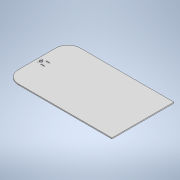
# Autodesk Inventor part: щиток
Saved by Autodesk Inventor 2021.1 (Build 251245010, 245A)
## iProperties
Created: 2023-04-14
Part Number: щиток
Material: Типовые
Document SubType Name: Modeling
Designer: User
Density: 1 g/cm^3
Appearance: По умолчанию
Author: User
Autodesk Inventor part; units mm, degrees
ref_plane "YZ Plane" through (0, 0, 0) normal (1, 0, 0) x (0, 1, 0)
ref_plane "XZ Plane" through (0, 0, 0) normal (0, 1, 0) x (-1, 0, 0)
ref_plane "XY Plane" through (0, 0, 0) normal (0, 0, 1) x (1, 0, 0)
sketch "Эскиз1" plane through (0, 0, 0) normal (0, 1, 0) x (-1, 0, 0)
  ellipse E0 centre (0, 0) end of major axis (0, -190) minor radius 325
  line L0 (0, 190) -> (-325, 190)
  line L1 (-325, 190) -> (-325, -190)
  line L2 (-325, -190) -> (0, -190)
  line L3 (0, -190) -> (0, 190)
  line L4 (0, 190) -> (325, 190)
  line L5 (325, 190) -> (325, -190)
  line L6 (325, -190) -> (0, -190)
  line L7 (0, -190) -> (0, 190)
  point P0 (0, -190)
  dimension "d0" = 325
  dimension "d1" = 190
  constraints: 16 end point, 4 horizontal, 4 parallel, 2 perpendicular, 2 vertical, 1 coincident, 1 vertical alignment, 2 other
extrude "Выдавливание1" add sketch "Эскиз1" along normal blind 6
fillet "Сопряжение1" radius 75 2 edges at (-325, 3, -190) (-325, 3, 190)
sketch "Эскиз2" plane through (0, 0, 0) normal (0, -1, 0) x (1, 0, 0)
  line L0 (-325, 0) -> (325, 0) construction
  line L1 (325, 190) -> (325, -190) projected
  line L2 (-325, 25) -> (-295, 14.0809)
  line L3 (-295, 14.0809) -> (97.2224, 27.7776)
  line L4 (97.2224, 27.7776) -> (125, 0)
  line L5 (-325, -115) -> (-325, 115) projected
  line L6 (-325, -25) -> (-295, -14.0809)
  line L7 (-295, -14.0809) -> (97.2224, -27.7776)
  line L8 (97.2224, -27.7776) -> (125, 0)
  line L9 (-325, 115) -> (-325, -115)
  line L10 (-260, 60) -> (-190, 60)
  line L11 (-190, 60) -> (-190, 130)
  line L12 (-190, 130) -> (-260, 130)
  line L13 (-260, 130) -> (-260, 60)
  line L14 (-190, 60) -> (-175.5025, 95)
  line L15 (-175.5025, 95) -> (-190, 130)
  line L16 (-218.335, 0) -> (-218.335, 60) construction
  line L17 (-250, 190) -> (325, 190) projected
  line L18 (-250, 190) -> (325, 190) projected
  line L19 (-250, 190) -> (-331.0569, 190) construction
  line L20 (-218.335, 130) -> (-218.335, 190) construction
  arc A0 (-250, 190) -> (-325, 115) centre (-250, 115) ccw projected
  line L21 (-175.5025, 51.7755) -> (-260, 130) construction
  line L22 (-260, 60) -> (-175.5025, 138.2245) construction
  circle A1 centre (-222.1933, 95) radius 14.4069 construction
  line L23 (-187.9955, 133) -> (-263, 133)
  line L24 (-263, 133) -> (-263, 57)
  line L25 (-263, 57) -> (-187.9955, 57)
  line L26 (-187.9955, 133) -> (-172.2553, 95)
  line L27 (-172.2553, 95) -> (-187.9955, 57)
  line L28 (-260, 95) -> (-253, 95)
  circle A2 centre (-253, 95) radius 5
  circle A3 centre (-253, 96.8516) radius 0.6666
  circle A4 centre (-253, 93.1484) radius 0.6666
  dimension "d5" = 45
  dimension "d8" = 133
  dimension "d9" = 25
  dimension "d10" = 70
  dimension "d11" = 30
  dimension "d12" = 135
  dimension "d13" = 70
  dimension "d15" = 60
  dimension "d16" = 3
  dimension "d17" = 3
  dimension "d20" = 7
  dimension "d21" = 10
  dimension "d27" = 200
  constraints: 50 end point, 9 point on line, 6 symmetric about line, 4 centre point, 4 equal length, 3 horizontal, 3 midpoint, 3 parallel, 3 perpendicular, 2 collinear, 1 coincident, 4 other
  measures "d5" angle of L4 L0
  measures "d8" angle of L4 L3
  measures "d9" distance from line of L2.start L0
  measures "d10" angle of L5 L2
  measures "d11" distance from line of L5 L2.end
  measures "d12" angle of L15 L14
  measures "d13" distance of L11.end L12.end
  measures "d15" distance from line of A0.centre L11
  measures "d16" distance between parallel lines of L26 L15
  measures "d17" distance between parallel lines of L23 L12
  measures "d20" distance from line of L13 L28.end
  measures "d21" diameter of A2
  measures "d27" distance from line of L1 L4.end
extrude "Выдавливание2" cut sketch "Эскиз2" against normal blind 0.5
sketch "Эскиз3" plane through (0, 0, 0) normal (0, -1, 0) x (1, 0, 0)
  line L0 (-295, -14.0809) -> (-325, -25) projected
  circle A0 centre (-300.125, 0) radius 8.5
  line L1 (97.2224, -27.7776) -> (-295, -14.0809) projected
  line L2 (-295, -14.0809) -> (-300.125, 0) construction
  circle A1 centre (-305.205, -14.48) radius 1.6
  line L3 (-325, -25) -> (-325, 25) projected
  line L4 (-325, 0) -> (327.0887, 0) construction
  line L5 (-308.505, -17.78) -> (-264.055, -17.78)
  line L6 (-264.055, -17.78) -> (-264.055, 17.78)
  line L7 (-264.055, 17.78) -> (-308.505, 17.78)
  line L8 (-308.505, 17.78) -> (-308.505, -17.78)
  line L9 (-264.055, -17.78) -> (-280.3762, 0) construction
  line L10 (-264.055, 17.78) -> (-280.3762, 0) construction
  line L11 (-264.055, 17.78) -> (-285.037, 17.78)
  line L12 (-285.037, 17.78) -> (-285.037, 14.418)
  line L13 (-285.037, 14.418) -> (-264.055, 14.418)
  line L14 (-264.055, 14.418) -> (-264.055, 17.78)
  line L15 (-285.037, -17.78) -> (-285.037, -14.418)
  line L16 (-285.037, -14.418) -> (-264.055, -14.418)
  circle A2 centre (-305.205, 14.48) radius 1.6
  point P0 (0, 0)
  point P1 (-308.505, 1.4232)
  point P2 (-308.505, -1.4232)
  dimension "d22" = 17
  dimension "d23" = 5.08
  dimension "d25" = 14.48
  dimension "d26" = 3.2
  dimension "d28" = 44.45
  dimension "d29" = 35.56
  dimension "d30" = 8.38
  dimension "d31" = 3.362
  dimension "d32" = 20.982
  constraints: 28 end point, 4 parallel, 4 perpendicular, 4 symmetric about line, 3 centre point, 2 horizontal, 2 point on line, 1 equal length, 1 midpoint, 1 other
  measures "d22" diameter of A0
  measures "d23" horizontal distance of A1.centre L2.end
  measures "d25" vertical distance of A1.centre L2.end
  measures "d26" diameter of A1
  measures "d28" distance of L6.end L7.end
  measures "d29" distance of L7.end L5.start
  measures "d30" distance from line of L8 L2.end
  measures "d31" distance between parallel lines of L11 L13
  measures "d32" distance between parallel lines of L6 L12
extrude "Выдавливание3" cut sketch "Эскиз3" against normal blind 14.48 contours L15 L16 L6 L1 | L1 L6 L5 L15 | L8 A0 | L13 L12 L7 L6 | A1 | A2 picked at (-298.3314, -3.5155)
equation "\"d33\" = d25"
